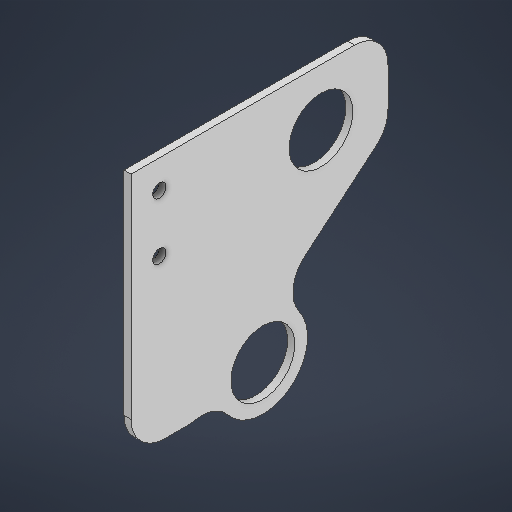
# Autodesk Inventor part: INSIDE_INTAKE_PLATE
Saved by Autodesk Inventor 2026.2 (Build 302298010, 298A)
## iProperties
Created: 2026-04-02
Part Number: INSIDE_INTAKE_PLATE
Material: Generic
Document SubType Name: Sheet Metal
Designer: 4aida
Density: 1 g/cm^3
Sheet Metal Rule: Default_mm
Appearance: Default
Author: 4aida
Autodesk Inventor part; units mm, degrees
ref_plane "YZ Plane" through (0, 0, 0) normal (1, 0, 0) x (0, 1, 0)
ref_plane "XZ Plane" through (0, 0, 0) normal (0, 1, 0) x (-1, 0, 0)
ref_plane "XY Plane" through (0, 0, 0) normal (0, 0, 1) x (1, 0, 0)
sketch "Sketch1" plane through (0, 0, 0) normal (1, 0, 0) x (0, 1, 0)
  line L0 (-39.3892, -115) -> (-110, -30.8494)
  line L1 (-110, -30.8494) -> (-110, 0)
  line L2 (-110, 0) -> (0, 0)
  line L3 (0, 0) -> (0, -115)
  line L4 (0, -115) -> (-39.3892, -115)
  line L5 (-110, -30.8494) -> (-119.38, 0) construction
  line L6 (-119.38, 0) -> (-110, 0) construction
  line L7 (-50.8, -25.4) -> (0, -25.4) construction
  line L8 (0, -25.4) -> (0, 0) construction
  line L9 (0, 0) -> (-50.8, 0) construction
  line L10 (-50.8, 0) -> (-50.8, -25.4) construction
  line L11 (-50.8, -25.4) -> (0, 0) construction
  line L12 (0, -25.4) -> (-50.8, 0) construction
  circle A0 centre (-12.7, -12.7) radius 3
  circle A1 centre (-38.1, -12.7) radius 3
  circle A2 centre (-102.5, -59) radius 14.2875
  circle A3 centre (-25.4, -85) radius 14.2875
  circle A4 centre (-102.5, -59) radius 20
  circle A5 centre (-25.4, -85) radius 30
  line L13 (-50.8, -100.9637) -> (-50.8, -69.0363)
  point P0 (-25.4, -12.7)
  point P1 (-25.4, -25.4)
  point P2 (-103.1519, -39.0106)
  point P3 (-82.9275, -63.1131)
  point P4 (-50.8, -85)
  dimension "d0" = 50
  dimension "d1" = 119.38
  dimension "d2" = 50.8
  dimension "d3" = 25.4
  dimension "d4" = 25.4
  dimension "d5" = 12.7
  dimension "d6" = 6
  dimension "d7" = 6
  dimension "d8" = 28.575
  dimension "d9" = 102.5
  dimension "d10" = 59
  dimension "d11" = 85
  dimension "d13" = 110
  dimension "d16" = 60
  dimension "d17" = 25.4
  dimension "d18" = 25.4
  dimension "d20" = 40
  measures "d0" angle of L0 L2
  measures "d1" distance from line of L3 L5.end
  measures "d2" distance of L7.start L7.end
  measures "d3" distance of L9.end L7.start
  measures "d4" distance of A1.centre A0.centre
  measures "d5" distance of point (-25.4, -12.7) A0.centre
  measures "d6" diameter of A0
  measures "d7" diameter of A1
  measures "d8" diameter of A2
  measures "d9" distance from line of A2.centre L3
  measures "d10" distance from line of L2 A2.centre
  measures "d11" distance from line of A3.centre L9
  measures "d13" distance between parallel lines of L3 L1
  measures "d16" diameter of A5
  measures "d17" distance from line of A3.centre L3
  measures "d18" distance of point (-50.8, -85) A3.centre
  measures "d20" diameter of A4
extrude "Plate1" add sketch "Sketch1" along normal blind 3.175 contours L0 A5 L4 | L0 A4 L1 L2 L3 A5 | A5 L13 L3 | A5 L3 L4 | A4 L0 A2 | L0 A2 A4 | A5 L13
fillet "Corner Round1" radius 15 6 edges at (1.5875, -82.9275, -63.1131) (1.5875, -103.1519, -39.0106) (1.5875, -110, -30.8494) (1.5875, -110, 0) (1.5875, 0, -115) (1.5875, -39.3892, -115)
equation "\"d5\" = 0.5 * d4"
equation "\"d7\" = d6"
equation "\"d14\" = Thickness"
equation "\"d18\" = d17"
equation "\"BendRadius\" = Thickness"
equation "\"BendReliefWidth\" = Thickness"
equation "\"BendReliefDepth\" = 0.5 * Thickness"
equation "\"CornerReliefSize\" = 4 * Thickness"
equation "\"MinimumRemnant\" = 2 * Thickness"
equation "\"TransitionRadius\" = BendRadius"
equation "\"JacobiRadiusSize\" = BendRadius"
equation "\"GapSize\" = Thickness"
equation "\"Thickness\" = 3.175"
body "Solid1"
